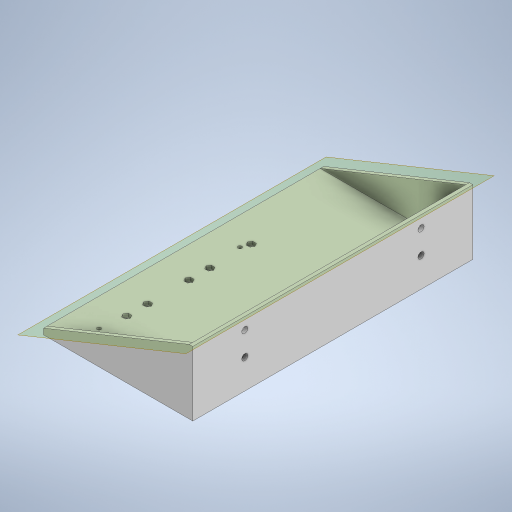
# Autodesk Inventor part: Soporte
Saved by Autodesk Inventor 2024 (Build 280153000, 153)
## iProperties
Created: 2024-01-17
Part Number: Soporte
Material: Generic
Document SubType Name: Modeling
Designer: juanp
Density: 1 g/cm^3
Appearance: Default
Author: juanp
Autodesk Inventor part; units mm, degrees
ref_plane "YZ Plane" through (0, 0, 0) normal (1, 0, 0) x (0, 1, 0)
ref_plane "XZ Plane" through (0, 0, 0) normal (0, 1, 0) x (-1, 0, 0)
ref_plane "XY Plane" through (0, 0, 0) normal (0, 0, 1) x (1, 0, 0)
sketch "Sketch1" plane through (0, 0, 0) normal (0, 1, 0) x (-1, 0, 0)
  line L0 (60.5, -116.25) -> (-60.5, -116.25)
  line L1 (-60.5, -116.25) -> (-60.5, 116.25)
  line L2 (-60.5, 116.25) -> (60.5, 116.25)
  line L3 (60.5, 116.25) -> (60.5, -116.25)
  line L4 (60.5, -116.25) -> (-60.5, 116.25) construction
  line L5 (-60.5, -116.25) -> (60.5, 116.25) construction
  line L6 (-40, 10.25) -> (-40, 60.25)
  line L7 (40, 10.25) -> (-40, 10.25)
  line L8 (40, 60.25) -> (40, 10.25)
  line L9 (-40, 60.25) -> (40, 60.25)
  circle A0 centre (37, 22) radius 1.75
  circle A1 centre (-37, 13.25) radius 1.75
  circle A2 centre (37, 57.25) radius 1.75
  circle A3 centre (-37, 57.25) radius 1.75
  circle A4 centre (37, -31) radius 1.75
  line L10 (40, -42.75) -> (-40, -42.75)
  circle A5 centre (-37, -39.75) radius 1.75
  circle A6 centre (37, 4.25) radius 1.75
  line L11 (40, 7.25) -> (40, -42.75)
  line L12 (-40, 7.25) -> (40, 7.25)
  circle A7 centre (-37, 4.25) radius 1.75
  line L13 (-40, -42.75) -> (-40, 7.25)
  circle A8 centre (37, 75) radius 1.75
  line L14 (40, 63.25) -> (-40, 63.25)
  circle A9 centre (-37, 66.25) radius 1.75
  circle A10 centre (37, 110.25) radius 1.75
  line L15 (40, 113.25) -> (40, 63.25)
  line L16 (-40, 113.25) -> (40, 113.25)
  circle A11 centre (-37, 110.25) radius 1.75
  line L17 (-40, 63.25) -> (-40, 113.25)
  line L18 (57.5, -45.75) -> (-57.5, -45.75)
  line L19 (-57.5, -45.75) -> (-57.5, -113.25)
  line L20 (-57.5, -113.25) -> (57.5, -113.25)
  line L21 (57.5, -113.25) -> (57.5, -45.75)
  line L22 (57.5, -45.75) -> (-57.5, -113.25) construction
  line L23 (-57.5, -45.75) -> (57.5, -113.25) construction
  line L24 (0, 113.25) -> (0, 113.2503) construction
  line L25 (63.5, 119.25) -> (-63.5, 119.25)
  line L26 (-63.5, 119.25) -> (-63.5, -119.25)
  line L27 (-63.5, -119.25) -> (63.5, -119.25)
  line L28 (63.5, -119.25) -> (63.5, 119.25)
  point P0 (0, 0)
  point P1 (0, -79.5)
  point P2 (0, -42.75)
  dimension "d6" = 3
  dimension "d7" = 3
  dimension "d8" = 3
  dimension "d9" = 3
  dimension "d10" = 3
  dimension "d11" = 11.75
  dimension "d12" = 3
  dimension "d13" = 3
  dimension "d14" = 50
  dimension "d15" = 80
  dimension "d16" = 3
  dimension "d17" = 3
  dimension "d18" = 3
  dimension "d19" = 3
  dimension "d20" = 3
  dimension "d21" = 11.75
  dimension "d22" = 3
  dimension "d23" = 3
  dimension "d24" = 50
  dimension "d25" = 80
  dimension "d26" = 3
  dimension "d27" = 3
  dimension "d28" = 3
  dimension "d29" = 3
  dimension "d30" = 3
  dimension "d31" = 11.75
  dimension "d32" = 3
  dimension "d33" = 3
  dimension "d34" = 50
  dimension "d35" = 80
  dimension "d36" = 3
  dimension "d37" = 3
  dimension "d38" = 67.5
  dimension "d39" = 115
  dimension "d43" = 3
  dimension "d44" = 3
  dimension "d46" = 3.5
  dimension "d47" = 3
  dimension "d48" = 3
  dimension "d49" = 3
  dimension "d50" = 3
  constraints: 58 end point, 12 centre point, 12 perpendicular, 11 equal radius, 6 midpoint, 6 parallel, 5 horizontal, 2 collinear, 1 point on line, 1 vertical, 3 other
  measures "d6" distance from line of L6 A1.centre
  measures "d7" distance from line of L6 A3.centre
  measures "d8" distance from line of L8 A0.centre
  measures "d9" distance from line of A2.centre L8
  measures "d10" distance from line of L9 A2.centre
  measures "d11" distance from line of L7 A0.centre
  measures "d12" distance from line of L9 A3.centre
  measures "d13" distance from line of L7 A1.centre
  measures "d14" distance of L7.end L9.start
  measures "d15" distance of L9.start L8.start
  measures "d16" distance from line of L13 A5.centre
  measures "d17" distance from line of L13 A7.centre
  measures "d18" distance from line of L11 A4.centre
  measures "d19" distance from line of A6.centre L11
  measures "d20" distance from line of L12 A6.centre
  measures "d21" distance from line of L10 A4.centre
  measures "d22" distance from line of L12 A7.centre
  measures "d23" distance from line of L10 A5.centre
  measures "d24" distance of L13.start L13.end
  measures "d25" distance of L13.end L11.start
  measures "d26" distance from line of L17 A9.centre
  measures "d27" distance from line of L17 A11.centre
  measures "d28" distance from line of L15 A8.centre
  measures "d29" distance from line of A10.centre L15
  measures "d30" distance from line of L16 A10.centre
  measures "d31" distance from line of L14 A8.centre
  measures "d32" distance from line of L16 A11.centre
  measures "d33" distance from line of L14 A9.centre
  measures "d34" distance of L17.start L17.end
  measures "d35" distance of L17.end L15.start
  measures "d36" distance between parallel lines of L9 L14
  measures "d37" distance between parallel lines of L12 L7
  measures "d38" distance of L19.end L18.end
  measures "d39" distance between parallel lines of L19 L21
  measures "d43" distance between parallel lines of L3 L21
  measures "d44" distance between parallel lines of L19 L1
  measures "d46" diameter of A10
  measures "d47" distance between parallel lines of L2 L16
  measures "d48" distance between parallel lines of L0 L20
  measures "d49" distance between parallel lines of L10 L18
  measures "d50" distance between parallel lines of L27 L0
extrude "Extrusion1" add sketch "Sketch1" along normal blind 5 contours L0 L1 L2 L3 | L6 L9 L8 L7 | L10 L13 L12 L11 | L14 L17 L16 L15 | L21 L20 L19 L18 | L28 L27 L26 L25
extrude "Extrusion2" add sketch "Sketch1" against normal blind 5 contours L28 L27 L26 L25
sketch "Sketch2" plane through (0, 0, 0) normal (0, -1, 0) x (1, 0, 0)
  line L0 (-39.6, -23.9821) -> (40.4, -23.9821) construction
  line L1 (40.4, -23.9821) -> (40.4, 96.0179) construction
  line L2 (40.4, 96.0179) -> (-39.6, 96.0179) construction
  line L3 (-39.6, 96.0179) -> (-39.6, -23.9821) construction
  line L4 (-39.6, -23.9821) -> (40.4, 96.0179) construction
  line L5 (40.4, -23.9821) -> (-39.6, 96.0179) construction
  line L6 (-48.6, -83.9821) -> (48.6, -83.9821) construction
  line L7 (48.6, -83.9821) -> (48.6, 114.5179) construction
  line L8 (48.6, 114.5179) -> (-48.6, 114.5179) construction
  line L9 (-48.6, 114.5179) -> (-48.6, -83.9821) construction
  line L10 (-48.6, -83.9821) -> (48.6, 114.5179) construction
  line L11 (48.6, -83.9821) -> (-48.6, 114.5179) construction
  circle A0 centre (-39.6, 96.0179) radius 1.65
  circle A1 centre (40.4, 96.0179) radius 1.65
  circle A2 centre (40.4, -23.9821) radius 1.65
  circle A3 centre (-39.6, -23.9821) radius 1.65
  line L12 (60.5, -116.25) -> (-60.5, -116.25) projected
  line L13 (0, -116.25) -> (0, 15.2679)
  point P0 (0.4, 36.0179)
  point P1 (-39.6, 36.0179)
  dimension "d61" = 80
  dimension "d62" = 120
  dimension "d63" = 97.2
  dimension "d64" = 198.5
  dimension "d65" = 9
  dimension "d66" = 60
  dimension "d67" = 3.3
  dimension "d70" = 131.518
  constraints: 26 end point, 6 midpoint, 4 centre point, 4 coincident, 4 parallel, 3 equal radius, 3 perpendicular, 1 horizontal
  measures "d61" distance of L3.start L2.start
  measures "d62" distance of L2.start L0.end
  measures "d63" distance of L9.start L7.end
  measures "d64" distance of L7.end L6.end
  measures "d65" distance from line of L9 point (-39.6, 36.018)
  measures "d66" distance between parallel lines of L6 L0
  measures "d67" diameter of A0
  measures "d70" distance of L13.start L13.end
extrude "Extrusion3" cut sketch "Sketch2" against normal blind 5
sketch "Sketch3" plane through (0, 5, 0) normal (0, 1, 0) x (1, 0, 0)
  line L0 (-63.5, -119.25) -> (63.5, -119.25) projected
  line L1 (63.5, 119.25) -> (-63.5, 119.25) projected
  line L2 (63.5, -119.25) -> (60.5, -119.25)
  line L3 (60.5, -119.25) -> (60.5, 119.25)
  line L4 (60.5, 119.25) -> (63.5, 119.25)
  line L5 (63.5, 119.25) -> (63.5, -119.25)
  point P0 (0, 0)
  dimension "d73" = 3
  constraints: 8 end point, 2 parallel, 1 horizontal, 1 perpendicular, 1 point on line
  measures "d73" distance between parallel lines of L5 L3
extrude "Extrusion4" add sketch "Sketch3" along normal blind 50
ref_plane "Work Plane1" through (60.5, 55, -119.25) normal (0.374, -0.9274, 0) x (0, 0, 1)
sketch "Sketch4" plane through (60.5, 55, -119.25) normal (0.374, -0.9274, 0) x (0, 0, 1)
  line L0 (0, 0) -> (238.5, 0) projected
  line L1 (0, 133.7012) -> (238.5, 133.7012) projected
  line L2 (238.5, 0) -> (235.5, 0)
  line L3 (235.5, 0) -> (235.5, 133.7012)
  line L4 (235.5, 133.7012) -> (238.5, 133.7012)
  line L5 (238.5, 133.7012) -> (238.5, 0)
  line L6 (0, -2.7823) -> (0, 0) projected
  line L7 (0, 0) -> (3, 0)
  line L8 (3, 0) -> (3, 133.7012)
  line L9 (3, 133.7012) -> (0, 133.7012)
  line L10 (0, 133.7012) -> (0, 0)
  point P0 (119.25, 76.6785)
  point P1 (0, 133.7012)
  point P2 (238.5, 133.7012)
  point P3 (235.5, 0)
  dimension "d76" = 3
  dimension "d77" = 3
  constraints: 16 end point, 4 parallel, 2 horizontal, 2 perpendicular, 2 point on line
  measures "d76" distance between parallel lines of L5 L3
  measures "d77" distance between parallel lines of L8 L10
extrude "Extrusion5" add sketch "Sketch4" along normal up to next contours L10 L1 L8 L0 | L3 L1 L5 L0
sketch "Sketch5" plane through (0, -5, 0) normal (0, -1, 0) x (1, 0, 0)
  line L0 (60.5, -116.25) -> (-60.5, -116.25) projected
  line L1 (-60.5, -116.25) -> (-60.5, 116.25) projected
  line L2 (-60.5, 116.25) -> (60.5, 116.25) projected
  line L3 (60.5, 116.25) -> (60.5, -116.25) projected
  line L4 (-63.5, -119.25) -> (63.5, -119.25) projected
  line L5 (63.5, -119.25) -> (63.5, 119.25) projected
  line L6 (63.5, 119.25) -> (-63.5, 119.25) projected
  line L7 (-63.5, 119.25) -> (-63.5, -119.25) projected
  point P0 (0, 0)
extrude "Extrusion6" cut sketch "Sketch5" against normal up to surface (5 mm away) contours L0 L1 L2 L3 | L7 L6 L5 L4
sketch "Sketch6" plane through (60.5, 5, -116.25) normal (-1, 0, 0) x (0, 0, 1)
  line L0 (235.5, 50) -> (-3, 50) projected
  line L1 (116.25, 50) -> (116.25, 40)
  line L2 (116.25, 40) -> (116.25, 20)
  line L3 (191.25, 20) -> (41.25, 20) construction
  line L4 (191.25, 40) -> (41.25, 40) construction
  line L5 (0, 0) -> (232.5, 0) projected
  circle A0 centre (191.25, 20) radius 2.65
  circle A1 centre (191.25, 40) radius 2.65
  circle A2 centre (41.25, 40) radius 2.65
  circle A3 centre (41.25, 20) radius 2.65
  point P0 (116.25, -5)
  dimension "d82" = 5.3
  dimension "d83" = 20
  dimension "d84" = 10
  dimension "d85" = 150
  constraints: 8 end point, 4 centre point, 4 coincident, 3 equal radius, 3 midpoint, 2 horizontal, 1 parallel, 1 point on line, 1 vertical
  measures "d82" diameter of A0
  measures "d83" distance between parallel lines of L3 L4
  measures "d84" distance of L1.start L1.end
  measures "d85" distance of L3.start L3.end
extrude "Extrusion7" cut sketch "Sketch6" against normal through all
sketch "Sketch7" plane through (0, 0, 0) normal (0, -1, 0) x (1, 0, 0)
  line L0 (-63.5, 119.25) -> (63.5, 119.25) projected
  line L1 (-63.5, -119.25) -> (-63.5, 119.25) projected
  line L2 (63.5, -119.25) -> (-63.5, -119.25) projected
  line L3 (63.5, 119.25) -> (63.5, -119.25) projected
  circle A0 centre (40.4, 96.0179) radius 1.65 projected
  circle A1 centre (40.4, -23.9821) radius 1.65 projected
  circle A2 centre (-39.6, 96.0179) radius 1.65 projected
  circle A3 centre (-39.6, -23.9821) radius 1.65 projected
  circle A4 centre (-37, 22) radius 1.75 projected
  circle A5 centre (37, 13.25) radius 1.75 projected
  circle A6 centre (-37, 57.25) radius 1.75 projected
  circle A7 centre (37, 57.25) radius 1.75 projected
  circle A8 centre (-37, -31) radius 1.75 projected
  circle A9 centre (-37, 4.25) radius 1.75 projected
  circle A10 centre (37, -39.75) radius 1.75 projected
  circle A11 centre (37, 4.25) radius 1.75 projected
  circle A12 centre (37, 66.25) radius 1.75 projected
  circle A13 centre (-37, 75) radius 1.75 projected
  circle A14 centre (-37, 110.25) radius 1.75 projected
  circle A15 centre (37, 110.25) radius 1.75 projected
  circle A16 centre (40.4, 96.0179) radius 5
  circle A17 centre (-39.6, 96.0179) radius 5
  circle A18 centre (-39.6, -23.9821) radius 5
  circle A19 centre (40.4, -23.9821) radius 5
  point P0 (0, 0)
  dimension "d88" = 10
  constraints: 4 centre point, 4 coincident, 3 equal radius
  measures "d88" diameter of A19
extrude "Extrusion8" cut sketch "Sketch7" against normal blind 3 contours A16 | A17 | A18 | A19
sketch "Sketch8" plane through (0, 5, 0) normal (0, 1, 0) x (1, 0, 0)
  circle A0 centre (40.4, -96.0179) radius 1.65 projected
  circle A1 centre (40.4, 23.9821) radius 1.65 projected
  circle A2 centre (-39.6, -96.0179) radius 1.65 projected
  circle A3 centre (-39.6, 23.9821) radius 1.65 projected
  circle A4 centre (-37, -22) radius 1.75 projected
  circle A5 centre (37, -13.25) radius 1.75 projected
  circle A6 centre (-37, -57.25) radius 1.75 projected
  circle A7 centre (37, -57.25) radius 1.75 projected
  circle A8 centre (-37, 31) radius 1.75 projected
  circle A9 centre (-37, -4.25) radius 1.75 projected
  circle A10 centre (37, 39.75) radius 1.75 projected
  circle A11 centre (37, -4.25) radius 1.75 projected
  circle A12 centre (37, -66.25) radius 1.75 projected
  circle A13 centre (-37, -75) radius 1.75 projected
  circle A14 centre (-37, -110.25) radius 1.75 projected
  circle A15 centre (37, -110.25) radius 1.75 projected
  line L0 (60.5, 116.25) -> (-63.5, 116.25) projected
  line L1 (-63.5, 116.25) -> (-63.5, -116.25) projected
  line L2 (-63.5, -116.25) -> (60.5, -116.25) projected
  line L3 (60.5, -116.25) -> (60.5, 116.25) projected
  line L4 (35.3979, 36.975) -> (33.7957, 39.75)
  line L5 (33.7957, 39.75) -> (35.3979, 42.525)
  line L6 (35.3979, 42.525) -> (38.6021, 42.525)
  line L7 (38.6021, 42.525) -> (40.2043, 39.75)
  line L8 (40.2043, 39.75) -> (38.6021, 36.975)
  line L9 (38.6021, 36.975) -> (35.3979, 36.975)
  line L10 (35.3979, -1.475) -> (38.6021, -1.475)
  line L11 (38.6021, -1.475) -> (40.2043, -4.25)
  line L12 (40.2043, -4.25) -> (38.6021, -7.025)
  line L13 (38.6021, -7.025) -> (35.3979, -7.025)
  line L14 (35.3979, -7.025) -> (33.7957, -4.25)
  line L15 (33.7957, -4.25) -> (35.3979, -1.475)
  line L16 (35.3979, -16.025) -> (33.7957, -13.25)
  line L17 (33.7957, -13.25) -> (35.3979, -10.475)
  line L18 (35.3979, -10.475) -> (38.6021, -10.475)
  line L19 (38.6021, -10.475) -> (40.2043, -13.25)
  line L20 (40.2043, -13.25) -> (38.6021, -16.025)
  line L21 (38.6021, -16.025) -> (35.3979, -16.025)
  line L22 (35.3979, -54.475) -> (38.6021, -54.475)
  line L23 (38.6021, -54.475) -> (40.2043, -57.25)
  line L24 (40.2043, -57.25) -> (38.6021, -60.025)
  line L25 (38.6021, -60.025) -> (35.3979, -60.025)
  line L26 (35.3979, -60.025) -> (33.7957, -57.25)
  line L27 (33.7957, -57.25) -> (35.3979, -54.475)
  line L28 (35.3979, -63.475) -> (38.6021, -63.475)
  line L29 (38.6021, -63.475) -> (40.2043, -66.25)
  line L30 (40.2043, -66.25) -> (38.6021, -69.025)
  line L31 (38.6021, -69.025) -> (35.3979, -69.025)
  line L32 (35.3979, -69.025) -> (33.7957, -66.25)
  line L33 (33.7957, -66.25) -> (35.3979, -63.475)
  line L34 (35.3979, -107.475) -> (38.6021, -107.475)
  line L35 (38.6021, -107.475) -> (40.2043, -110.25)
  line L36 (40.2043, -110.25) -> (38.6021, -113.025)
  line L37 (38.6021, -113.025) -> (35.3979, -113.025)
  line L38 (35.3979, -113.025) -> (33.7957, -110.25)
  line L39 (33.7957, -110.25) -> (35.3979, -107.475)
  line L40 (-38.6021, 33.775) -> (-35.3979, 33.775)
  line L41 (-35.3979, 33.775) -> (-33.7957, 31)
  line L42 (-33.7957, 31) -> (-35.3979, 28.225)
  line L43 (-35.3979, 28.225) -> (-38.6021, 28.225)
  line L44 (-38.6021, 28.225) -> (-40.2043, 31)
  line L45 (-40.2043, 31) -> (-38.6021, 33.775)
  line L46 (-38.6021, -1.475) -> (-35.3979, -1.475)
  line L47 (-35.3979, -1.475) -> (-33.7957, -4.25)
  line L48 (-33.7957, -4.25) -> (-35.3979, -7.025)
  line L49 (-35.3979, -7.025) -> (-38.6021, -7.025)
  line L50 (-38.6021, -7.025) -> (-40.2043, -4.25)
  line L51 (-40.2043, -4.25) -> (-38.6021, -1.475)
  line L52 (-38.6021, -19.225) -> (-35.3979, -19.225)
  line L53 (-35.3979, -19.225) -> (-33.7957, -22)
  line L54 (-33.7957, -22) -> (-35.3979, -24.775)
  line L55 (-35.3979, -24.775) -> (-38.6021, -24.775)
  line L56 (-38.6021, -24.775) -> (-40.2043, -22)
  line L57 (-40.2043, -22) -> (-38.6021, -19.225)
  line L58 (-38.6021, -54.475) -> (-35.3979, -54.475)
  line L59 (-35.3979, -54.475) -> (-33.7957, -57.25)
  line L60 (-33.7957, -57.25) -> (-35.3979, -60.025)
  line L61 (-35.3979, -60.025) -> (-38.6021, -60.025)
  line L62 (-38.6021, -60.025) -> (-40.2043, -57.25)
  line L63 (-40.2043, -57.25) -> (-38.6021, -54.475)
  line L64 (-40.2043, -75) -> (-38.6021, -72.225)
  line L65 (-38.6021, -72.225) -> (-35.3979, -72.225)
  line L66 (-35.3979, -72.225) -> (-33.7957, -75)
  line L67 (-33.7957, -75) -> (-35.3979, -77.775)
  line L68 (-35.3979, -77.775) -> (-38.6021, -77.775)
  line L69 (-38.6021, -77.775) -> (-40.2043, -75)
  line L70 (-38.6021, -107.475) -> (-35.3979, -107.475)
  line L71 (-35.3979, -107.475) -> (-33.7957, -110.25)
  line L72 (-33.7957, -110.25) -> (-35.3979, -113.025)
  line L73 (-35.3979, -113.025) -> (-38.6021, -113.025)
  line L74 (-38.6021, -113.025) -> (-40.2043, -110.25)
  line L75 (-40.2043, -110.25) -> (-38.6021, -107.475)
  point P0 (0, 0)
  dimension "d91" = 5.55
  constraints: 144 end point, 12 coincident, 12 horizontal, 11 equal length, 156 other
  measures "d91" distance between parallel lines of L31 L28
extrude "Extrusion9" cut sketch "Sketch8" against normal blind 3 contours A0 | A1 | A2 | A3 | A4 | A5 | A6 | A7 | A8 | A9 | A10 | A11 | A12 | A13 | A14 | A15 | L4 L5 L6 L7 L8 L9 | L10 L11 L12 L13 L14 L15 | L16 L17 L18 L19 L20 L21 | L22 L23 L24 L25 L26 L27 | L28 L29 L30 L31 L32 L33 | L34 L35 L36 L37 L38 L39 | L40 L41 L42 L43 L44 L45 | L46 L47 L48 L49 L50 L51 | L52 L53 L54 L55 L56 L57 | L58 L59 L60 L61 L62 L63 | L64 L65 L66 L67 L68 L69 | L70 L71 L72 L73 L74 L75
body "Solid1"
